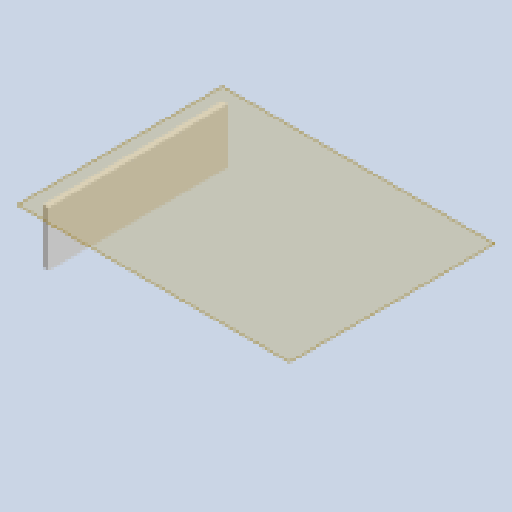
# Autodesk Inventor part: стенка
Saved by Autodesk Inventor 2024.2 (Build 282272000, 272)
## iProperties
Created: 2025-12-09
Part Number: стенка
Material: Типовые
Document SubType Name: Modeling
Designer: katya_notebook
Mass: 65.1748 g
Surface Area: 247.334 cm^2
Volume: 65.1748 cm^3
Density: 1 g/cm^3
Appearance: По умолчанию
Author: katya_notebook
Autodesk Inventor part; units mm, degrees
ref_plane "YZ Plane" through (0, 0, 0) normal (1, 0, 0) x (0, 1, 0)
ref_plane "XZ Plane" through (0, 0, 0) normal (0, 1, 0) x (-1, 0, 0)
ref_plane "XY Plane" through (0, 0, 0) normal (0, 0, 1) x (1, 0, 0)
ref_plane "РабПлоскость1" through (-475.2675, -216.9886, 379.0883) normal (0, 1, 0) x (-1, 0, 0)
sketch "Эскиз1" plane through (-475.2675, -216.9886, 379.0883) normal (0, 1, 0) x (-1, 0, 0)
  line L0 (135, 97.5) -> (129, 97.5)
  line L1 (129, 97.5) -> (129, -97.5)
  line L2 (129, -97.5) -> (135, -97.5)
  line L3 (135, -97.5) -> (135, 97.5)
  line L4 (135, -97.5) -> (135, 97.5) projected
  line L5 (135, 97.5) -> (62.5237, 97.5) projected
  line L6 (62.5237, -97.5) -> (135, -97.5) projected
  point P0 (-475.2675, -379.0883)
  dimension "d0" = 0
  dimension "d1" = 6
  dimension "d2" = 0
  dimension "d3" = 0
  constraints: 8 end point, 2 parallel, 1 horizontal, 1 perpendicular
  measures "d0" distance between parallel lines of L4 L3
  measures "d1" distance of L0.start L0.end
  measures "d2" distance between parallel lines of L6 L2
  measures "d3" distance between parallel lines of L0 L5
ref_plane "РабПлоскость2" through (-610.2675, -276.6936, 277.5883) normal (0, 1, 0) x (0, 0, 1)
extrude "Выдавливание1" add sketch "Эскиз1" against normal up to surface (59.705 mm away)
sketch "Эскиз2" plane through (-610.2675, -216.9886, 281.5883) normal (-1, 0, 0) x (0, 0, 1)
  line L0 (0, -4) -> (195, -4) projected
  line L1 (195, 0) -> (195, -59.705) projected
  line L2 (0, 0) -> (195, 0) projected
  line L3 (0, 0) -> (0, -59.705) projected
  point P0 (-281.5883, 216.9886)
extrude "Выдавливание2" cut sketch "Эскиз2" against normal blind 10
sketch "Эскиз3" plane through (-610.2675, -276.6936, 281.5883) normal (-1, 0, 0) x (0, 0, 1)
  line L0 (195, 0) -> (0, 0) projected
  line L1 (175, 0) -> (155, 0)
  line L2 (155, 0) -> (155, -5)
  line L3 (155, -5) -> (175, -5)
  line L4 (175, -5) -> (175, 0)
  line L5 (195, 55.705) -> (195, 0) projected
  line L6 (135, 0) -> (115, 0)
  line L7 (115, 0) -> (115, -5)
  line L8 (115, -5) -> (135, -5)
  line L9 (135, -5) -> (135, 0)
  line L10 (20, 0) -> (40, 0)
  line L11 (40, 0) -> (40, -4)
  line L12 (40, -4) -> (20, -4)
  line L13 (20, -4) -> (20, 0)
  line L14 (60, 0) -> (80, 0)
  line L15 (80, 0) -> (80, -4)
  line L16 (80, -4) -> (60, -4)
  line L17 (60, -4) -> (60, 0)
  line L18 (97.5, 27.8525) -> (226.4185, 27.8525)
  line L19 (195, 55.705) -> (0, 55.705)
  line L20 (175, 55.705) -> (155, 55.705)
  line L21 (155, 55.705) -> (155, 60.705)
  line L22 (155, 60.705) -> (175, 60.705)
  line L23 (175, 60.705) -> (175, 55.705)
  line L24 (135, 55.705) -> (115, 55.705)
  line L25 (115, 55.705) -> (115, 60.705)
  line L26 (115, 60.705) -> (135, 60.705)
  line L27 (135, 60.705) -> (135, 55.705)
  line L28 (20, 55.705) -> (40, 55.705)
  line L29 (40, 55.705) -> (40, 59.705)
  line L30 (40, 59.705) -> (20, 59.705)
  line L31 (20, 59.705) -> (20, 55.705)
  line L32 (60, 55.705) -> (80, 55.705)
  line L33 (80, 55.705) -> (80, 59.705)
  line L34 (80, 59.705) -> (60, 59.705)
  line L35 (60, 59.705) -> (60, 55.705)
  point P0 (-281.5883, 276.6936)
  point P1 (40, 55.705)
  point P2 (80, 55.705)
  point P3 (40, 0)
  point P4 (80, 0)
  point P5 (115, 55.705)
  point P6 (155, 55.705)
  point P7 (115, 0)
  point P8 (155, 0)
  dimension "d8" = 5
  dimension "d9" = 20
  dimension "d10" = 20
  dimension "d11" = 20
  dimension "d12" = 20
  dimension "d13" = 4
  dimension "d14" = 20
  dimension "d15" = 20
  dimension "d16" = 20
  dimension "d17" = 20
  constraints: 68 end point, 17 symmetric about line, 8 parallel, 8 point on line, 5 horizontal, 4 perpendicular
  measures "d8" distance of L3.end L1.start
  measures "d9" distance of L2.end L3.end
  measures "d10" distance of L0.start L1.start
  measures "d11" distance of L7.end L8.end
  measures "d12" distance of L1.end L6.start
  measures "d13" distance of L10.end L11.end
  measures "d14" distance of L11.end L12.end
  measures "d15" distance of L10.start L0.end
  measures "d16" distance of L15.end L16.end
  measures "d17" distance of L14.start L10.end
extrude "Выдавливание3" add sketch "Эскиз3" against normal blind 6
sketch "Эскиз4" plane through (-610.2675, -276.6936, 281.5883) normal (-1, 0, 0) x (0, 0, 1)
  point P0 (-281.5883, 276.6936)
sketch "Эскиз5" plane through (-610.2675, -276.6936, 281.5883) normal (-1, 0, 0) x (0, 0, 1)
  point P0 (-281.5883, 276.6936)
sketch "Эскиз6" plane through (-610.2675, -276.6936, 281.5883) normal (-1, 0, 0) x (0, 0, 1)
  line L0 (111.125, 6.5) -> (104.625, 6.5)
  line L1 (104.625, 6.5) -> (104.625, 9.5)
  line L2 (104.625, 9.5) -> (111.125, 9.5)
  line L3 (111.125, 9.5) -> (111.125, 6.5)
  line L4 (115, 0) -> (115, -5) projected
  line L5 (100.75, 6.5) -> (94.25, 6.5)
  line L6 (94.25, 6.5) -> (94.25, 9.5)
  line L7 (94.25, 9.5) -> (100.75, 9.5)
  line L8 (100.75, 9.5) -> (100.75, 6.5)
  line L9 (90.375, 6.5) -> (83.875, 6.5)
  line L10 (83.875, 6.5) -> (83.875, 9.5)
  line L11 (83.875, 9.5) -> (90.375, 9.5)
  line L12 (90.375, 9.5) -> (90.375, 6.5)
  line L13 (111.125, 8) -> (104.625, 8)
  line L14 (115, 0) -> (80, 0) projected
  line L15 (106.125, 16) -> (109.625, 16)
  line L16 (109.625, 16) -> (109.625, 0)
  line L17 (109.625, 0) -> (106.125, 0)
  line L18 (106.125, 0) -> (106.125, 16)
  line L19 (106.125, 16) -> (109.625, 0) construction
  line L20 (109.625, 16) -> (106.125, 0) construction
  line L21 (100.75, 8) -> (94.25, 8)
  line L22 (97.5, 6.5) -> (97.5, 9.5)
  line L23 (90.375, 8) -> (83.875, 8)
  line L24 (87.125, 6.5) -> (87.125, 9.5)
  line L25 (95.75, 16) -> (99.25, 16)
  line L26 (99.25, 16) -> (99.25, 0)
  line L27 (99.25, 0) -> (95.75, 0)
  line L28 (95.75, 0) -> (95.75, 16)
  line L29 (95.75, 16) -> (99.25, 0) construction
  line L30 (99.25, 16) -> (95.75, 0) construction
  line L31 (85.375, 16) -> (88.875, 16)
  line L32 (88.875, 16) -> (88.875, 0)
  line L33 (88.875, 0) -> (85.375, 0)
  line L34 (85.375, 0) -> (85.375, 16)
  line L35 (85.375, 16) -> (88.875, 0) construction
  line L36 (88.875, 16) -> (85.375, 0) construction
  line L37 (148.25, 6.5) -> (141.75, 6.5)
  line L38 (141.75, 6.5) -> (141.75, 9.5)
  line L39 (141.75, 9.5) -> (148.25, 9.5)
  line L40 (148.25, 9.5) -> (148.25, 6.5)
  line L41 (148.25, 8) -> (141.75, 8)
  line L42 (143.25, 16) -> (146.75, 16)
  line L43 (146.75, 16) -> (146.75, 0)
  line L44 (146.75, 0) -> (143.25, 0)
  line L45 (143.25, 0) -> (143.25, 16)
  line L46 (143.25, 16) -> (146.75, 0) construction
  line L47 (146.75, 16) -> (143.25, 0) construction
  line L48 (155, 0) -> (155, -5) projected
  line L49 (53.25, 6.5) -> (46.75, 6.5)
  line L50 (46.75, 6.5) -> (46.75, 9.5)
  line L51 (46.75, 9.5) -> (53.25, 9.5)
  line L52 (53.25, 9.5) -> (53.25, 6.5)
  line L53 (53.25, 8) -> (46.75, 8)
  line L54 (48.25, 16) -> (51.75, 16)
  line L55 (51.75, 16) -> (51.75, 0)
  line L56 (51.75, 0) -> (48.25, 0)
  line L57 (48.25, 0) -> (48.25, 16)
  line L58 (48.25, 16) -> (51.75, 0) construction
  line L59 (51.75, 16) -> (48.25, 0) construction
  line L60 (60, 0) -> (60, -4) projected
  line L61 (195, 55.705) -> (195, 0) projected
  line L62 (195, 27.8525) -> (88.875, 27.8525)
  line L63 (111.125, 49.205) -> (104.625, 49.205)
  line L64 (104.625, 49.205) -> (104.625, 46.205)
  line L65 (104.625, 46.205) -> (111.125, 46.205)
  line L66 (111.125, 46.205) -> (111.125, 49.205)
  line L67 (115, 55.705) -> (115, 60.705)
  line L68 (100.75, 49.205) -> (94.25, 49.205)
  line L69 (94.25, 49.205) -> (94.25, 46.205)
  line L70 (94.25, 46.205) -> (100.75, 46.205)
  line L71 (100.75, 46.205) -> (100.75, 49.205)
  line L72 (90.375, 49.205) -> (83.875, 49.205)
  line L73 (83.875, 49.205) -> (83.875, 46.205)
  line L74 (83.875, 46.205) -> (90.375, 46.205)
  line L75 (90.375, 46.205) -> (90.375, 49.205)
  line L76 (111.125, 47.705) -> (104.625, 47.705)
  line L77 (115, 55.705) -> (80, 55.705)
  line L78 (106.125, 39.705) -> (109.625, 39.705)
  line L79 (109.625, 39.705) -> (109.625, 55.705)
  line L80 (109.625, 55.705) -> (106.125, 55.705)
  line L81 (106.125, 55.705) -> (106.125, 39.705)
  line L82 (106.125, 39.705) -> (109.625, 55.705) construction
  line L83 (109.625, 39.705) -> (106.125, 55.705) construction
  line L84 (100.75, 47.705) -> (94.25, 47.705)
  line L85 (97.5, 49.205) -> (97.5, 46.205)
  line L86 (90.375, 47.705) -> (83.875, 47.705)
  line L87 (87.125, 49.205) -> (87.125, 46.205)
  line L88 (95.75, 39.705) -> (99.25, 39.705)
  line L89 (99.25, 39.705) -> (99.25, 55.705)
  line L90 (99.25, 55.705) -> (95.75, 55.705)
  line L91 (95.75, 55.705) -> (95.75, 39.705)
  line L92 (95.75, 39.705) -> (99.25, 55.705) construction
  line L93 (99.25, 39.705) -> (95.75, 55.705) construction
  line L94 (85.375, 39.705) -> (88.875, 39.705)
  line L95 (88.875, 39.705) -> (88.875, 55.705)
  line L96 (88.875, 55.705) -> (85.375, 55.705)
  line L97 (85.375, 55.705) -> (85.375, 39.705)
  line L98 (85.375, 39.705) -> (88.875, 55.705) construction
  line L99 (88.875, 39.705) -> (85.375, 55.705) construction
  line L100 (146.75, 55.705) -> (143.25, 55.705)
  line L101 (146.75, 39.705) -> (146.75, 55.705)
  line L102 (146.75, 39.705) -> (143.25, 55.705) construction
  line L103 (143.25, 39.705) -> (146.75, 55.705) construction
  line L104 (143.25, 55.705) -> (143.25, 39.705)
  line L105 (141.75, 49.205) -> (141.75, 46.205)
  line L106 (148.25, 49.205) -> (141.75, 49.205)
  line L107 (148.25, 46.205) -> (148.25, 49.205)
  line L108 (141.75, 46.205) -> (148.25, 46.205)
  line L109 (148.25, 47.705) -> (141.75, 47.705)
  line L110 (143.25, 39.705) -> (146.75, 39.705)
  line L111 (155, 55.705) -> (155, 60.705)
  line L112 (51.75, 55.705) -> (48.25, 55.705)
  line L113 (51.75, 39.705) -> (51.75, 55.705)
  line L114 (51.75, 39.705) -> (48.25, 55.705) construction
  line L115 (48.25, 39.705) -> (51.75, 55.705) construction
  line L116 (48.25, 55.705) -> (48.25, 39.705)
  line L117 (46.75, 49.205) -> (46.75, 46.205)
  line L118 (53.25, 49.205) -> (46.75, 49.205)
  line L119 (53.25, 46.205) -> (53.25, 49.205)
  line L120 (46.75, 46.205) -> (53.25, 46.205)
  line L121 (53.25, 47.705) -> (46.75, 47.705)
  line L122 (48.25, 39.705) -> (51.75, 39.705)
  line L123 (60, 55.705) -> (60, 59.705)
  point P0 (-281.5883, 276.6936)
  point P1 (115, -2.5)
  point P2 (107.875, 11.6549)
  point P3 (107.875, 8)
  point P4 (97.5, 8)
  point P5 (87.125, 8)
  point P6 (149.0518, 14.6563)
  point P7 (145, 8)
  point P8 (155, -2.5)
  point P9 (49.2049, 25.9501)
  point P10 (50, 8)
  point P11 (60, -2)
  point P12 (48.25, 9.5)
  point P13 (48.25, 6.5)
  point P14 (51.75, 6.5)
  point P15 (51.75, 9.5)
  point P16 (88.875, 9.5)
  point P17 (85.375, 9.5)
  point P18 (85.375, 6.5)
  point P19 (85.375, 0)
  point P20 (88.875, 6.5)
  point P21 (95.75, 6.5)
  point P22 (95.75, 0)
  point P23 (99.25, 6.5)
  point P24 (99.25, 9.5)
  point P25 (95.75, 9.5)
  point P26 (106.125, 6.5)
  point P27 (106.125, 0)
  point P28 (109.625, 6.5)
  point P29 (109.625, 9.5)
  point P30 (106.125, 9.5)
  point P31 (143.25, 6.5)
  point P32 (146.75, 6.5)
  point P33 (146.75, 9.5)
  point P34 (143.25, 9.5)
  point P35 (115, 58.205)
  point P36 (107.875, 44.0501)
  point P37 (107.875, 47.705)
  point P38 (97.5, 47.705)
  point P39 (87.125, 47.705)
  point P40 (145, 47.705)
  point P41 (149.0518, 41.0486)
  point P42 (155, 58.205)
  point P43 (50, 47.705)
  point P44 (60, 57.705)
  point P45 (51.75, 46.205)
  point P46 (51.75, 49.205)
  point P47 (48.25, 49.205)
  point P48 (48.25, 46.205)
  point P49 (88.875, 46.205)
  point P50 (88.875, 49.205)
  point P51 (85.375, 55.705)
  point P52 (85.375, 49.205)
  point P53 (85.375, 46.205)
  point P54 (99.25, 46.205)
  point P55 (99.25, 49.205)
  point P56 (95.75, 49.205)
  point P57 (95.75, 46.205)
  point P58 (106.125, 49.205)
  point P59 (106.125, 46.205)
  point P60 (109.625, 46.205)
  point P61 (109.625, 49.205)
  point P62 (143.25, 49.205)
  point P63 (143.25, 46.205)
  point P64 (146.75, 46.205)
  point P65 (146.75, 49.205)
  dimension "d20" = 6.5
  dimension "d21" = 3
  dimension "d22" = 3.875
  dimension "d23" = 6.5
  dimension "d24" = 3
  dimension "d25" = 3.875
  dimension "d26" = 6.5
  dimension "d27" = 3
  dimension "d28" = 3.875
  dimension "d29" = 8
  dimension "d30" = 3.5
  dimension "d31" = 3.5
  dimension "d32" = 3.5
  dimension "d33" = 6.5
  dimension "d34" = 3
  dimension "d35" = 3.5
  dimension "d36" = 8.25
  dimension "d37" = 6.5
  dimension "d38" = 3
  dimension "d39" = 3.5
  dimension "d40" = 8.25
  constraints: 238 end point, 71 symmetric about line, 33 midpoint, 20 parallel, 12 perpendicular, 11 horizontal, 6 point on line, 4 collinear
  measures "d20" distance of L0.start L0.end
  measures "d21" distance of L0.end L1.end
  measures "d22" horizontal distance of L13.start point (115, -2.5)
  measures "d23" distance of L5.start L5.end
  measures "d24" distance of L5.end L6.end
  measures "d25" distance of L7.end L1.end
  measures "d26" distance of L9.start L9.end
  measures "d27" distance of L9.end L10.end
  measures "d28" distance of L6.end L11.end
  measures "d29" distance from line of L14 point (107.875, 8)
  measures "d30" distance of L16.end L17.end
  measures "d31" distance of L27.end L26.end
  measures "d32" distance of L33.end L32.end
  measures "d33" distance of L37.start L38.start
  measures "d34" distance of L38.start L38.end
  measures "d35" distance of L44.start L44.end
  measures "d36" distance from line of L43 point (155, -2.5)
  measures "d37" distance of L49.start L50.start
  measures "d38" distance of L50.start L50.end
  measures "d39" distance of L56.start L56.end
  measures "d40" distance from line of L55 point (60, -2)
extrude "Выдавливание4" cut sketch "Эскиз6" against normal blind 6
